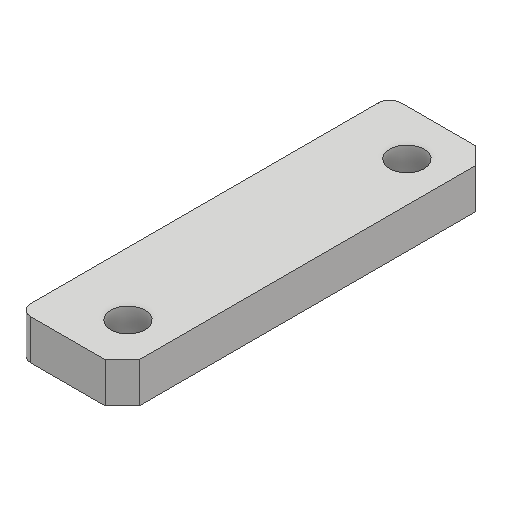
# Autodesk Inventor part: 3DP_ABS_E3D_Titan_Mounting_Plate_Spacer
Saved by Autodesk Inventor 2026.1 (Build 301233000, 233)
## iProperties
Created: 2017-07-28
Part Number: 3DP_ABS_E3D_Titan_Mounting_Plate_Spacer
Material: Ogólny
Document SubType Name: Modeling
Designer: Andrzej
Density: 1 g/cm^3
Appearance: Domyślna
Author: Andrzej
Autodesk Inventor part; units mm, degrees
ref_plane "YZ Plane" through (0, 0, 0) normal (1, 0, 0) x (0, 1, 0)
ref_plane "XZ Plane" through (0, 0, 0) normal (0, 1, 0) x (-1, 0, 0)
ref_plane "XY Plane" through (0, 0, 0) normal (0, 0, 1) x (1, 0, 0)
sketch "Szkic1" plane through (0, 0, 0) normal (0, 0, 1) x (1, 0, 0)
  circle A0 centre (9.199, -9.5538) radius 1.5
  circle A1 centre (9.199, 14.8462) radius 1.5
  line L0 (-3.801, -13.5538) -> (-5.301, -12.0538)
  line L1 (-3.801, -13.5538) -> (11.199, -13.5538)
  line L2 (12.699, -12.0538) -> (11.199, -13.5538)
  line L3 (12.699, 17.3462) -> (12.699, -12.0538)
  line L4 (11.199, 18.8462) -> (12.699, 17.3462)
  line L5 (11.199, 18.8462) -> (-3.801, 18.8462)
  line L6 (-5.301, 17.3462) -> (-3.801, 18.8462)
  line L7 (-5.301, 17.3462) -> (-5.301, -12.0538)
  circle A2 centre (0.699, -7.3538) radius 1.5
  circle A3 centre (0.699, 12.6462) radius 1.5
  line L8 (3.699, 18.8462) -> (3.699, -13.5538)
  point P0 (0, 0)
  point P1 (0, 0)
  dimension "d0" = 9
  constraints: 18 end point, 4 centre point, 2 midpoint
  measures "d0" distance between parallel lines of L3 L8
extrude "Wyciągnięcie proste1" add sketch "Szkic1" along normal blind 3.5 contours L8 L5 L4 L3 L2 L1
fillet "Zaokrąglenie1" radius 1 2 edges at (3.699, -13.5538, 1.75) (3.699, 18.8462, 1.75)
